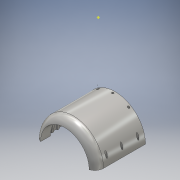
# Autodesk Inventor part: UR5 Joint base connection2
Saved by Autodesk Inventor 2016 (Build 200138000, 138)
## iProperties
Created: 2017-12-24
Part Number: UR5 Joint base connection2
Material: Aluminum 6061-AHC
Document SubType Name: Modeling
Designer: kornbot
Density: 2.7 g/cm^3
Appearance: Aluminum - Dark
Author: kornbot
Autodesk Inventor part; units mm, degrees
sketch "Sketch1" plane through (0, 0, 0) normal (0, 0, 1) x (1, 0, 0)
  line L0 (0, 0) -> (0, 80)
  line L1 (0, 80) -> (-43.275, 80)
  line L2 (-43.275, 80) -> (-46.275, 80)
  line L3 (-46.275, 80) -> (-43.275, 80)
  line L4 (-43.275, 80) -> (-43.275, 0)
  line L5 (-43.275, 0) -> (-46.275, 0)
  line L6 (-46.275, 80) -> (-48.275, 80)
  line L7 (-48.275, 80) -> (-43.275, 80)
  line L8 (-43.275, 80) -> (-43.275, 0)
  line L9 (-43.275, 0) -> (-48.275, 0)
  line L10 (-48.275, 0) -> (-48.275, 80)
  line L11 (-43.275, 0) -> (-43.275, 25)
  line L12 (-43.275, 25) -> (-43.275, 23.7)
  line L13 (-43.275, 25) -> (-43.275, 29.3)
  line L14 (-43.275, 29.3) -> (-43.275, 32.3)
  line L15 (-43.275, 23.7) -> (-43.275, 20.7)
  line L16 (-43.275, 20.7) -> (-41.525, 20.7)
  line L17 (-43.275, 23.7) -> (-41.525, 23.7)
  line L18 (-41.525, 23.7) -> (-41.525, 20.7)
  line L19 (-41.525, 20.7) -> (-43.275, 20.7)
  line L20 (-43.275, 20.7) -> (-43.275, 23.7)
  line L21 (-43.275, 32.3) -> (-41.525, 32.3)
  line L22 (-43.275, 32.3) -> (-41.2868, 32.3)
  line L23 (-41.2868, 32.3) -> (-41.2868, 29.3)
  line L24 (-41.2868, 29.3) -> (-43.275, 29.3)
  line L25 (-43.275, 29.3) -> (-43.275, 32.3)
  line L26 (-43.275, 0) -> (-38.651, 0)
  line L27 (-43.275, 20.7) -> (-43.275, 15.7)
  line L28 (-43.275, 15.7) -> (-38.651, 15.7)
  line L29 (-38.651, 15.7) -> (-38.651, 0)
  dimension "d1" = 80
  dimension "d2" = 43.275
  dimension "d3" = 3
  dimension "d4" = 2
  dimension "d5" = 25
  dimension "d6" = 1.3
  dimension "d7" = 4.3
  dimension "d8" = 3
  dimension "d9" = 3
  dimension "d10" = 1.75
  dimension "d11" = 1.75
  dimension "d12" = 4.624
  dimension "d13" = 5
  constraints: 60 end point, 10 horizontal, 7 parallel, 6 perpendicular, 6 point on line, 1 vertical
  measures "d1" distance of L0.start L0.end
  measures "d2" distance of L0.end L1.end
  measures "d3" distance of L1.end L2.end
  measures "d4" distance of L2.end L6.end
  measures "d5" distance of L4.end L11.end
  measures "d6" distance of L11.end L12.end
  measures "d7" distance of L11.end L13.end
  measures "d8" distance of L13.end L14.end
  measures "d9" distance of L12.end L15.end
  measures "d10" distance of L15.end L16.end
  measures "d11" distance of L14.end L21.end
  measures "d12" distance of L4.end L26.end
  measures "d13" distance of L19.end L27.end
revolve "Revolution1" add sketch "Sketch1" angle 180 about axis through (0, 0, 0) along (0, 1, 0)
sketch "Sketch2" plane through (48.275, 0, 0) normal (0, 0, -1) x (-1, 0, 0)
  line L0 (9.624, 15.7) -> (5, 15.7) projected
  line L1 (5, 15.7) -> (5, 0)
  line L2 (96.55, 0) -> (0, 0) projected
  line L3 (0, 79.5517) -> (5, 0)
  line L4 (0, 80) -> (0, 0) projected
  line L5 (5, 79.5517) -> (0, 0)
  line L6 (0, 80) -> (0, 0)
  line L7 (5, 32.3) -> (5, 80) projected
  line L8 (2.5, 39.7758) -> (2.5, 19.7758)
  line L9 (2.5, 39.7758) -> (2.5, 69.7758)
  circle A0 centre (2.5, 19.7758) radius 1.5
  circle A1 centre (2.5, 69.7758) radius 1.5
  line L10 (2.5, 69.7758) -> (96.55, 69.7758)
  line L11 (2.5, 19.7758) -> (96.55, 20.7)
  line L12 (91.7692, 15.7) -> (91.7692, 0)
  line L13 (91.55, 32.3) -> (91.55, 80) projected
  line L14 (91.55, 80) -> (96.55, 0)
  line L15 (96.55, 0) -> (91.7692, 0)
  line L16 (96.55, 80) -> (96.55, 0) projected
  line L17 (91.7692, 0) -> (96.55, 80)
  line L18 (94.1596, 40) -> (94.1596, 70)
  circle A2 centre (94.1596, 70) radius 1.5
  line L19 (94.1596, 40) -> (93.9807, 37.0053)
  line L20 (94.1596, 40) -> (94.1596, 10)
  circle A3 centre (94.1596, 20.6765) radius 1.5
  point P0 (48.275, 0)
  dimension "d15" = 20
  dimension "d16" = 30
  dimension "d17" = 3
  dimension "d19" = 3
  dimension "d20" = 30
  dimension "d21" = 3
  dimension "d22" = 3
  dimension "d23" = 30
  dimension "d24" = 3
  constraints: 30 end point, 7 point on line, 4 centre point, 3 coincident, 3 parallel, 2 midpoint, 2 vertical, 1 collinear, 1 horizontal, 1 perpendicular
  measures "d15" distance of L8.start L8.end
  measures "d16" distance of L8.start L9.end
  measures "d17" diameter of A0
  measures "d19" diameter of A1
  measures "d20" distance of L18.start L18.end
  measures "d21" diameter of A2
  measures "d22" distance of L18.start L19.end
  measures "d23" distance of L18.start L20.end
  measures "d24" diameter of A3
extrude "Extrusion1" cut sketch "Sketch2" against normal blind 80 contours A3 L20 L11 L14 | L14 L11 A3 | A3 L11 L17 | L17 L11 L20 A3 | L14 A3 L11 | L11 L20 A3 L14 | A0 L5 L8 L11 L3 | L3 L11 A0 | L17 A3 L20 L11 | L11 A3 L17 | A0 L5 | L11 L8 A0 L3 | L3 A0 L11 | A2 L18 L10 | L10 A2 | L18 A2 L10 | A1 L10 L9 | L9 L10 A1
fillet "Fillet1" radius 14 1 edges at (0, 0, 48.275)
sketch "Sketch3" plane through (48.275, 80, 0) normal (0, 0, -1) x (-1, 0, 0)
  line L0 (2.4582, -60.3516) -> (2.4582, -9.8777)
  circle A0 centre (94.1596, -59.3235) radius 1.5 projected
  line L1 (94.1596, -9.8777) -> (94.1596, -59.3235)
  circle A1 centre (2.5, -10.2242) radius 1.5 projected
  line L2 (2.5, -10.2242) -> (2.4582, -35.8591)
  line L3 (2.4582, -35.8591) -> (94.1596, -35.8591)
  circle A2 centre (2.4582, -35.8591) radius 1.5
  circle A3 centre (94.1596, -35.8591) radius 1.5
  point P0 (48.275, -80)
  dimension "d28" = 25.635
  dimension "d29" = 3
  dimension "d30" = 3
  constraints: 8 end point, 2 centre point, 2 coincident, 2 point on line, 2 vertical, 1 horizontal
  measures "d28" distance of L2.start L2.end
  measures "d29" diameter of A2
  measures "d30" diameter of A3
extrude "Extrusion2" cut sketch "Sketch3" against normal blind 89.5 contours A2 L0 | L0 L3 A2 | L0 A2 L3 | A3 L1 | L1 L3 A3 | L1 A3 L3
ref_plane "Work Plane1" through (0, 40, 48.275) normal (0, 0, -1) x (-1, 0, 0)
sketch "Sketch4" plane through (-43.275, 80, 0) normal (0, 0, -1) x (-1, 0, 0)
  line L0 (-91.55, 0) -> (-91.55, -66.7015) projected
  line L1 (-91.55, 0) -> (-91.55, -7.7757)
  line L2 (-91.55, -7.7757) -> (5, -7.7757)
  line L3 (5, -7.7757) -> (5, 0)
  line L4 (0, 0) -> (-86.55, 0) projected
  line L5 (5, 0) -> (5, -66.7015) projected
  circle A0 centre (2.6096, -10) radius 1.5 projected
  circle A1 centre (-68.3306, -3.74) radius 1.5
  circle A2 centre (-43.275, -3.8878) radius 1.5
  circle A3 centre (-20.1965, -4.2625) radius 1.5
  point P0 (-43.275, -80)
  dimension "d33" = 3
  dimension "d35" = 3
  constraints: 6 end point, 3 centre point, 1 parallel, 1 point on line
  measures "d33" diameter of A1
  measures "d35" diameter of A3
extrude "Extrusion3" add sketch "Sketch4" against normal blind 141 contours A1 | A2 | A3
sketch "Sketch5" plane through (25.0556, 76.26, 141) normal (0, 0, 1) x (1, 0, 0)
  circle A0 centre (0, 0) radius 1.5 projected
  circle A1 centre (0, 0) radius 1.5
  circle A2 centre (-48.135, -0.5154) radius 1.5071
  circle A3 centre (-25.0556, -0.1515) radius 1.55
  point P0 (-25.0556, -76.26)
  dimension "d38" = 3.1
  constraints: 3 centre point, 1 coincident
  measures "d38" diameter of A3
extrude "Extrusion4" cut sketch "Sketch5" against normal blind 204
ref_plane "Work Plane2" through (-23.0785, 74.2375, 141) normal (0.0005956, -0.9999998, 0) x (0.9999998, 0.0005956, 0)
sketch "Sketch6" plane through (-48.275, 80, 0) normal (0, 1, 0) x (1, 0, 0)
  line L0 (-26.6471, -154.7697) -> (72.0573, -154.7697)
  line L1 (72.0573, -154.7697) -> (72.0573, -48.9374)
  line L2 (72.0573, -48.9374) -> (-26.6471, -48.9374)
  line L3 (-26.6471, -48.9374) -> (-26.6471, -154.7697)
  point P0 (48.275, 0)
  constraints: 8 end point, 2 parallel, 1 horizontal, 1 perpendicular
extrude "Extrusion5" cut sketch "Sketch6" against normal blind 167.25
sketch "Sketch7" plane through (-23.0785, 74.2375, 141) normal (0.0005956, -0.9999998, 0) x (0.9999998, 0.0005956, 0)
  point P0 (23.0343, -141)
ref_plane "Work Plane3" through (43.275, 0, 0) normal (-1, 0, 0) x (0, 1, 0)
sketch "Sketch9" plane through (0, 40, 48.275) normal (0, 0, -1) x (-1, 0, 0)
  circle A0 centre (22.9079, 35.8253) radius 1.6138
  point P0 (0, -40)
  constraints: 1 centre point
extrude "Extrusion7" cut sketch "Sketch9" along normal blind 48.75
body "Solid1"
